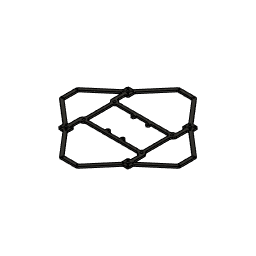
CarbonFiberBoard v13 (Autodesk Fusion 360 design; units mm, degrees)
Autodesk Fusion 360 part; units mm, degrees
sketch "草图1" plane through (0, 0, 0) normal (0, 0, 1) x (1, 0, 0)
  line L0 (42.5, 42.5) -> (-42.5, 42.5) construction
  line L1 (-42.5, 42.5) -> (-42.5, -42.5) construction
  line L2 (-42.5, -42.5) -> (42.5, -42.5) construction
  line L3 (42.5, -42.5) -> (42.5, 42.5) construction
  line L4 (42.5, 42.5) -> (-42.5, -42.5) construction
  line L5 (-42.5, 42.5) -> (42.5, -42.5) construction
  circle A0 centre (-42.5, 42.5) radius 2.25
  circle A1 centre (-45.682, 45.682) radius 1.05
  circle A2 centre (-45.682, 39.318) radius 1.05
  circle A3 centre (-39.318, 39.318) radius 1.05
  circle A4 centre (-39.318, 45.682) radius 1.05
  line L6 (0, 55) -> (0, -50) construction
  line L7 (-50, 0) -> (50, 0) construction
  circle A5 centre (45.682, 39.318) radius 1.05
  circle A6 centre (42.5, 42.5) radius 2.25
  circle A7 centre (39.318, 39.318) radius 1.05
  circle A8 centre (39.318, 45.682) radius 1.05
  circle A9 centre (45.682, 45.682) radius 1.05
  circle A10 centre (-45.682, -39.318) radius 1.05
  circle A11 centre (-45.682, -45.682) radius 1.05
  circle A12 centre (-42.5, -42.5) radius 2.25
  circle A13 centre (-39.318, -45.682) radius 1.05
  circle A14 centre (-39.318, -39.318) radius 1.05
  circle A15 centre (39.318, -45.682) radius 1.05
  circle A16 centre (45.682, -45.682) radius 1.05
  circle A17 centre (42.5, -42.5) radius 2.25
  circle A18 centre (39.318, -39.318) radius 1.05
  circle A19 centre (45.682, -39.318) radius 1.05
  line L8 (39.5, 21) -> (-39.5, 21) construction
  line L9 (-39.5, 21) -> (-39.5, -21) construction
  line L10 (-39.5, -21) -> (39.5, -21) construction
  line L11 (39.5, -21) -> (39.5, 21) construction
  line L12 (39.5, 21) -> (-39.5, -21) construction
  line L13 (-39.5, 21) -> (39.5, -21) construction
  circle A20 centre (-39.5, 21) radius 1.6
  circle A21 centre (39.5, 21) radius 1.6
  circle A22 centre (-39.5, -21) radius 1.6
  circle A23 centre (39.5, -21) radius 1.6
  line L14 (-35.9031, 22.75) -> (35.9031, 22.75)
  line L15 (-35.9031, 19.25) -> (35.9031, 19.25)
  line L16 (-41.25, 17.4031) -> (-41.25, -17.4031)
  line L17 (-37.75, 17.4031) -> (-37.75, -17.4031)
  line L18 (37.75, 17.4031) -> (37.75, -17.4031)
  line L19 (41.25, 17.4031) -> (41.25, -17.4031)
  line L20 (-35.9031, -19.25) -> (35.9031, -19.25)
  line L21 (-35.9031, -22.75) -> (35.9031, -22.75)
  line L22 (-40.5, 37) -> (-40.5, 24.873)
  line L23 (-42.7, 18.6) -> (-44.5, 21)
  line L24 (-44.5, 21) -> (-44.5, 37)
  line L25 (-38.5, 48) -> (-46.5, 48)
  line L26 (-48, 46.5) -> (-48, 38.5)
  line L27 (-37, 38.5) -> (-37, 46.5)
  line L28 (-37, 48) -> (-48, 37) construction
  line L29 (-48, 48) -> (-37, 37) construction
  arc A24 (-46.5, 48) -> (-48, 46.5) centre (-46.5, 46.5) ccw
  arc A25 (-48, 38.5) -> (-46.5, 37) centre (-46.5, 38.5) ccw
  arc A26 (-38.5, 37) -> (-37, 38.5) centre (-38.5, 38.5) ccw
  arc A27 (-37, 46.5) -> (-38.5, 48) centre (-38.5, 46.5) ccw
  line L30 (-46.5, 37) -> (-44.5, 37)
  line L31 (-40.5, 37) -> (-38.5, 37)
  arc A28 (-35.9031, 22.75) -> (-40.5, 24.873) centre (-39.5, 21) ccw
  arc A29 (-42.7, 18.6) -> (-41.25, 17.4031) centre (-39.5, 21) ccw
  arc A30 (48, 46.5) -> (46.5, 48) centre (46.5, 46.5) ccw
  line L32 (38.5, 48) -> (46.5, 48)
  arc A31 (38.5, 48) -> (37, 46.5) centre (38.5, 46.5) ccw
  line L33 (37, 38.5) -> (37, 46.5)
  line L34 (48, 46.5) -> (48, 38.5)
  arc A32 (46.5, 37) -> (48, 38.5) centre (46.5, 38.5) ccw
  line L35 (46.5, 37) -> (44.5, 37)
  line L36 (40.5, 37) -> (38.5, 37)
  arc A33 (37, 38.5) -> (38.5, 37) centre (38.5, 38.5) ccw
  line L37 (40.5, 37) -> (40.5, 24.873)
  line L38 (44.5, 21) -> (44.5, 37)
  line L39 (42.7, 18.6) -> (44.5, 21)
  line L40 (-46.5, -37) -> (-44.5, -37)
  arc A34 (-46.5, -37) -> (-48, -38.5) centre (-46.5, -38.5) ccw
  line L41 (-48, -46.5) -> (-48, -38.5)
  arc A35 (-48, -46.5) -> (-46.5, -48) centre (-46.5, -46.5) ccw
  line L42 (-38.5, -48) -> (-46.5, -48)
  arc A36 (-38.5, -48) -> (-37, -46.5) centre (-38.5, -46.5) ccw
  line L43 (-37, -38.5) -> (-37, -46.5)
  arc A37 (-37, -38.5) -> (-38.5, -37) centre (-38.5, -38.5) ccw
  line L44 (-40.5, -37) -> (-38.5, -37)
  line L45 (-40.5, -37) -> (-40.5, -24.873)
  line L46 (-44.5, -21) -> (-44.5, -37)
  line L47 (-42.7, -18.6) -> (-44.5, -21)
  line L48 (40.5, -37) -> (40.5, -24.873)
  line L49 (40.5, -37) -> (38.5, -37)
  arc A38 (38.5, -37) -> (37, -38.5) centre (38.5, -38.5) ccw
  line L50 (37, -38.5) -> (37, -46.5)
  arc A39 (37, -46.5) -> (38.5, -48) centre (38.5, -46.5) ccw
  line L51 (38.5, -48) -> (46.5, -48)
  arc A40 (46.5, -48) -> (48, -46.5) centre (46.5, -46.5) ccw
  line L52 (48, -46.5) -> (48, -38.5)
  arc A41 (48, -38.5) -> (46.5, -37) centre (46.5, -38.5) ccw
  line L53 (46.5, -37) -> (44.5, -37)
  line L54 (44.5, -21) -> (44.5, -37)
  line L55 (42.7, -18.6) -> (44.5, -21)
  arc A42 (41.25, 17.4031) -> (42.7, 18.6) centre (39.5, 21) ccw
  arc A43 (40.5, 24.873) -> (35.9031, 22.75) centre (39.5, 21) ccw
  arc A44 (-41.25, -17.4031) -> (-42.7, -18.6) centre (-39.5, -21) ccw
  arc A45 (-40.5, -24.873) -> (-35.9031, -22.75) centre (-39.5, -21) ccw
  arc A46 (35.9031, -22.75) -> (40.5, -24.873) centre (39.5, -21) ccw
  arc A47 (42.7, -18.6) -> (41.25, -17.4031) centre (39.5, -21) ccw
  arc A48 (37.75, -17.4031) -> (35.9031, -19.25) centre (39.5, -21) ccw
  arc A49 (35.9031, 19.25) -> (37.75, 17.4031) centre (39.5, 21) ccw
  arc A50 (-37.75, 17.4031) -> (-35.9031, 19.25) centre (-39.5, 21) ccw
  arc A51 (-35.9031, -19.25) -> (-37.75, -17.4031) centre (-39.5, -21) ccw
  point P0 (-42.5, 42.5)
  dimension "d1" = 85
  dimension "d2" = 85
  dimension "d3" = 4.5
  dimension "d4" = 2.1
  dimension "d5" = 4.5
  dimension "d7" = 360
  dimension "d9" = 79
  dimension "d10" = 42
  dimension "d11" = 3.2
  dimension "d12" = 8
  dimension "d13" = 8
  dimension "d14" = 8
  dimension "d15" = 8
  dimension "d16" = 3.5
  dimension "d17" = 3.5
  dimension "d18" = 2
  dimension "d19" = 2
  dimension "d20" = 11
  dimension "d21" = 11
  dimension "d22" = 1.5
  constraint horizontal L0
  constraint perpendicular L0 L1
  constraint parallel L0 L2
  constraint parallel L1 L3
  constraint coincident L4 origin
  constraint coincident L5 origin
  constraint coincident P0 L0.end
  constraint coincident L5 A1.centre
  constraint vertical L6
  constraint horizontal L7
  constraint symmetric A0 L6 A6
  constraint symmetric A1 L6 A9
  constraint symmetric A2 L6 A5
  constraint symmetric A3 L6 A7
  constraint symmetric A4 L6 A8
  constraint symmetric A0 L7 A12
  constraint symmetric A1 L7 A11
  constraint symmetric A2 L7 A10
  constraint symmetric A3 L7 A14
  constraint symmetric A4 L7 A13
  constraint symmetric L7 A5 A19
  constraint symmetric L7 A6 A17
  constraint symmetric L7 A7 A18
  constraint symmetric L7 A8 A15
  constraint symmetric L7 A9 A16
  constraint horizontal L8
  constraint perpendicular L8 L9
  constraint parallel L8 L10
  constraint parallel L9 L11
  constraint coincident L12 origin
  constraint coincident L13 origin
  constraint coincident L8.end L9.start
  constraint symmetric L6 A20 A21
  constraint symmetric L7 A20 A22
  constraint symmetric L7 A21 A23
  constraint concentric A20 A28
  constraint concentric A21 A42
  constraint concentric A22 A44
  constraint concentric A23 A46
  constraint parallel L8 L14
  constraint coincident L15.start A28
  constraint coincident L15.end A42
  constraint parallel L8 L15
  constraint symmetric L8 L14 L15
  constraint parallel L9 L16
  constraint coincident L17.start A28
  constraint parallel L9 L17
  constraint symmetric L6 L16.start L19.start
  constraint symmetric L6 L16.end L19.end
  constraint symmetric L6 L17.start L18.start
  constraint symmetric L6 L17.end L18.end
  constraint symmetric L7 L14.start L21.start
  constraint symmetric L7 L14.end L21.end
  constraint symmetric L7 L15.start L20.start
  constraint symmetric L7 L15.end L20.end
  constraint vertical L22
  constraint coincident L23.start A28
  constraint vertical L24
  constraint tangent L23 A28
  constraint horizontal L25
  constraint perpendicular L25 L26
  constraint parallel L25 L30
  constraint parallel L26 L27
  constraint coincident L28 P0
  constraint coincident L29 P0
  constraint coincident L29.start L26
  constraint coincident L29.start L25
  constraint tangent L26 A24
  constraint tangent L25 A24
  constraint coincident L28.end L26
  constraint coincident L28.end L30
  constraint tangent L26 A25
  constraint tangent A25 L30
  constraint equal A24 A25
  constraint coincident L29.end L30
  constraint coincident L29.end L27
  constraint tangent A26 L30
  constraint tangent L27 A26
  constraint equal A24 A26
  constraint coincident L28.start L27
  constraint coincident L28.start L25
  constraint tangent L27 A27
  constraint tangent L25 A27
  constraint equal A24 A27
  constraint coincident L22.start L30
  constraint collinear L30 L31
  constraint concentric A28 A29
  constraint symmetric L6 L22.start L36.start
  constraint symmetric L6 L22.end L37.end
  constraint symmetric L6 L23.start L39.start
  constraint symmetric L6 L23.end L38.start
  constraint symmetric L6 L24.end L35.end
  constraint symmetric L6 L26.start A30.start
  constraint symmetric L6 L25.end A30.end
  constraint symmetric L6 A24 A30
  constraint symmetric L6 L26.end L34.end
  constraint symmetric L6 A25.end A32.start
  constraint symmetric L6 A25 A32
  constraint symmetric L6 A26.start L36.end
  constraint symmetric L6 L27.start L33.start
  constraint symmetric L6 A26 A33
  constraint symmetric L6 L27.end A31.end
  constraint symmetric L6 L25.start L32.start
  constraint symmetric L6 A27 A31
  constraint symmetric L7 L22.start L44.start
  constraint symmetric L7 L22.end L45.end
  constraint symmetric L7 L23.start L47.start
  constraint symmetric L7 L23.end L46.start
  constraint symmetric L7 L24.end L40.end
  constraint symmetric L7 L26.start L41.start
  constraint symmetric L7 L25.end A35.end
  constraint symmetric L7 A24 A35
  constraint symmetric L7 L26.end A34.end
  constraint symmetric L7 A25.end L40.start
  constraint symmetric L7 A25 A34
  constraint symmetric L7 A26.start A37.end
  constraint symmetric L7 L27.start L43.start
  constraint symmetric L7 A26 A37
  constraint symmetric L7 L27.end A36.end
  constraint symmetric L7 L25.start L42.start
  constraint symmetric L7 A27 A36
  constraint symmetric L7 A30.end L51.end
  constraint symmetric L7 A30.start A40.end
  constraint symmetric L7 A30 A40
  constraint symmetric L7 L32.start A39.end
  constraint symmetric L7 A31.end L50.end
  constraint symmetric L7 A31 A39
  constraint symmetric L7 L33.start A38.end
  constraint symmetric L7 L34.end L52.end
  constraint symmetric L7 A32.start A41.end
  constraint symmetric L7 A32 A41
  constraint symmetric L7 L35.end L53.end
  constraint symmetric L7 L36.start L48.start
  constraint symmetric L7 L36.end L49.end
  constraint symmetric L7 A33 A38
  constraint symmetric L7 L37.end L48.end
  constraint symmetric L7 L38.start L54.start
  constraint symmetric L7 L39.start L55.start
  constraint concentric A42 A43
  constraint concentric A44 A45
  constraint concentric A46 A47
  constraint coincident L10.end L11.start
  constraint coincident L8.start L11.end
  constraint coincident L9.end L10.start
  measures "d1" distance of L0.start P0
  measures "d2" distance of L0 L2
  measures "d3" diameter of A0
  measures "d4" diameter of A1
  measures "d5" distance of P0 A1.centre
  measures "d9" distance of L8.start L8.end
  measures "d10" distance of L8 L10
  measures "d11" diameter of A20
  measures "d12" diameter of A28
  measures "d13" diameter of A42
  measures "d14" diameter of A44
  measures "d15" diameter of A46
  measures "d16" distance of L14 L15
  measures "d17" distance of L16 L17
  measures "d18" distance of L1 L22
  measures "d19" distance of L1 L24
  measures "d20" distance of L26 L27
  measures "d21" distance of L25 L30
  measures "d22" radius of A24
extrude "拉伸1" add sketch "草图1" along normal blind 2
fillet "圆角1" radius 1 8 edges at (-44.5, -37, 1) (-40.5, -37, 1) (44.5, -37, 1) (40.5, -37, 1) (-44.5, 37, 1) (40.5, 37, 1) (44.5, 37, 1) (-40.5, 37, 1)
fillet "圆角2" radius 3 4 edges at (-44.5, 21, 1) (-44.5, -21, 1) (44.5, -21, 1) (44.5, 21, 1)
fillet "圆角3" radius 3 4 edges at (41.25, -17.4031, 1) (41.25, 17.4031, 1) (-41.25, -17.4031, 1) (-41.25, 17.4031, 1)
fillet "圆角4" radius 2 4 edges at (-40.5, -24.873, 1) (-40.5, 24.873, 1) (40.5, 24.873, 1) (40.5, -24.873, 1)
fillet "圆角5" radius 2 4 edges at (35.9031, -22.75, 1) (-35.9031, -22.75, 1) (-35.9031, 22.75, 1) (35.9031, 22.75, 1)
sketch "草图3" plane through (0, 0, 0) normal (0, 0, 1) x (1, 0, 0)
  line L0 (10, 17.5) -> (-10, 17.5) construction
  line L1 (-10, 17.5) -> (-10, -17.5) construction
  line L2 (-10, -17.5) -> (10, -17.5) construction
  line L3 (10, -17.5) -> (10, 17.5) construction
  line L4 (10, 17.5) -> (-10, -17.5) construction
  line L5 (-10, 17.5) -> (10, -17.5) construction
  circle A0 centre (-10, 17.5) radius 1
  circle A1 centre (10, 17.5) radius 1
  circle A2 centre (-10, -17.5) radius 1
  circle A3 centre (10, -17.5) radius 1
  line L6 (-7.5, 17.5) -> (-7.5, 19.5)
  arc A4 (-7.5, 19.5) -> (-12.5, 19.5) centre (-10, 19.5) ccw
  line L7 (-12.5, 19.5) -> (-12.5, 17.5)
  arc A5 (-12.5, 17.5) -> (-7.5, 17.5) centre (-10, 17.5) ccw
  line L8 (-10, 17.5) -> (-10, 19.5) construction
  line L9 (0, 0) -> (0, 8.2439) construction
  line L10 (0, 0) -> (4, 0) construction
  arc A6 (7.5, 17.5) -> (12.5, 17.5) centre (10, 17.5) ccw
  line L11 (12.5, 19.5) -> (12.5, 17.5)
  arc A7 (12.5, 19.5) -> (7.5, 19.5) centre (10, 19.5) ccw
  line L12 (7.5, 17.5) -> (7.5, 19.5)
  arc A8 (-7.5, -17.5) -> (-12.5, -17.5) centre (-10, -17.5) ccw
  line L13 (-12.5, -19.5) -> (-12.5, -17.5)
  arc A9 (-12.5, -19.5) -> (-7.5, -19.5) centre (-10, -19.5) ccw
  line L14 (-7.5, -17.5) -> (-7.5, -19.5)
  line L15 (7.5, -17.5) -> (7.5, -19.5)
  arc A10 (7.5, -19.5) -> (12.5, -19.5) centre (10, -19.5) ccw
  line L16 (12.5, -19.5) -> (12.5, -17.5)
  arc A11 (12.5, -17.5) -> (7.5, -17.5) centre (10, -17.5) ccw
  dimension "d50" = 20
  dimension "d51" = 35
  dimension "d52" = 2
  dimension "d53" = 2
  dimension "d54" = 2
  dimension "d55" = 2
  dimension "d56" = 5
  dimension "d57" = 2
  constraint horizontal L0
  constraint perpendicular L0 L1
  constraint parallel L0 L2
  constraint parallel L1 L3
  constraint coincident L4 L9.start
  constraint coincident L5 L9.start
  constraint coincident L9.start L10.start
  constraint coincident L0.end L1.start
  constraint coincident L0.start L3.end
  constraint coincident L1.end L2.start
  constraint coincident L2.end L3.start
  constraint tangent L6 A4
  constraint tangent A4 L7
  constraint parallel L6 L7
  constraint tangent L7 A5
  constraint tangent L6 A5
  constraint parallel L1 L8
  constraint parallel L3 L9
  constraint perpendicular L9 L10
  constraint symmetric L6.start L9 A6.start
  constraint symmetric L6.end L9 A7.end
  constraint symmetric A4.end L9 L11.start
  constraint symmetric L7.end L9 A6.end
  constraint symmetric A4 L9 A7
  constraint symmetric A5 L9 A6
  constraint symmetric L6.start L10 A8.start
  constraint symmetric L6.end L10 A9.end
  constraint symmetric A4.end L10 L13.start
  constraint symmetric L7.end L10 A8.end
  constraint symmetric A4 L10 A9
  constraint symmetric A5 L10 A8
  constraint symmetric L10 A6.end L16.end
  constraint symmetric L10 A6.start L15.start
  constraint symmetric L10 A6 A11
  constraint symmetric L10 L11.start A10.end
  constraint symmetric L10 A7.end L15.end
  constraint symmetric L10 A7 A10
  measures "d50" distance of L1 L3
  measures "d51" distance of L0 L2
  measures "d52" diameter of A0
  measures "d53" diameter of A1
  measures "d54" diameter of A2
  measures "d55" diameter of A3
  measures "d56" distance of L6 L7
  measures "d57" distance of L0.end A4.centre
extrude "拉伸3" add sketch "草图3" along normal blind 2
sketch "草图5" plane through (0, 0, 2) normal (0, 0, 1) x (-1, 0, 0)
  circle A0 centre (-10, 17.5) radius 1
  line L0 (-7.5, 19.25) -> (7.5, 19.25)
  line L1 (7.5, 19.25) -> (7.5, 17.5)
  arc A1 (7.5, 17.5) -> (12.5, 17.5) centre (10, 17.5) ccw
  line L2 (12.5, 17.5) -> (12.5, 19.25)
  line L3 (12.5, 19.25) -> (35.9031, 19.25)
  arc A2 (35.9031, 19.25) -> (37.75, 17.4031) centre (39.5, 21) ccw
  line L4 (37.75, 17.4031) -> (37.75, -17.4031)
  arc A3 (37.75, -17.4031) -> (35.9031, -19.25) centre (39.5, -21) ccw
  line L5 (35.9031, -19.25) -> (12.5, -19.25)
  line L6 (12.5, -19.25) -> (12.5, -17.5)
  arc A4 (12.5, -17.5) -> (7.5, -17.5) centre (10, -17.5) ccw
  line L7 (7.5, -17.5) -> (7.5, -19.25)
  line L8 (7.5, -19.25) -> (-7.5, -19.25)
  line L9 (-7.5, -19.25) -> (-7.5, -17.5)
  arc A5 (-7.5, -17.5) -> (-12.5, -17.5) centre (-10, -17.5) ccw
  line L10 (-12.5, -17.5) -> (-12.5, -19.25)
  line L11 (-12.5, -19.25) -> (-35.9031, -19.25)
  arc A6 (-35.9031, -19.25) -> (-37.75, -17.4031) centre (-39.5, -21) ccw
  line L12 (-37.75, -17.4031) -> (-37.75, 17.4031)
  arc A7 (-37.75, 17.4031) -> (-35.9031, 19.25) centre (-39.5, 21) ccw
  line L13 (-35.9031, 19.25) -> (-12.5, 19.25)
  line L14 (-12.5, 19.25) -> (-12.5, 17.5)
  arc A8 (-12.5, 17.5) -> (-7.5, 17.5) centre (-10, 17.5) ccw
  line L15 (-7.5, 17.5) -> (-7.5, 19.25)
  circle A9 centre (10, -17.5) radius 1
  circle A10 centre (10, 17.5) radius 1
  circle A11 centre (-10, -17.5) radius 1
  circle A12 centre (39.318, -45.682) radius 1.05
  circle A13 centre (-45.682, -39.318) radius 1.05
  circle A14 centre (45.682, 39.318) radius 1.05
  circle A15 centre (45.682, 45.682) radius 1.05
  circle A16 centre (42.5, 42.5) radius 2.25
  circle A17 centre (39.318, 45.682) radius 1.05
  circle A18 centre (39.318, 39.318) radius 1.05
  circle A19 centre (45.682, -45.682) radius 1.05
  circle A20 centre (-39.318, -45.682) radius 1.05
  circle A21 centre (-39.318, -39.318) radius 1.05
  circle A22 centre (42.5, -42.5) radius 2.25
  circle A23 centre (45.682, -39.318) radius 1.05
  circle A24 centre (39.318, -39.318) radius 1.05
  circle A25 centre (-42.5, -42.5) radius 2.25
  circle A26 centre (-45.682, -45.682) radius 1.05
  circle A27 centre (39.5, 21) radius 1.6
  circle A28 centre (-39.5, 21) radius 1.6
  circle A29 centre (39.5, -21) radius 1.6
  circle A30 centre (-39.5, -21) radius 1.6
  circle A31 centre (-45.682, 39.318) radius 1.05
  circle A32 centre (-39.318, 39.318) radius 1.05
  circle A33 centre (-39.318, 45.682) radius 1.05
  circle A34 centre (-45.682, 45.682) radius 1.05
  circle A35 centre (-42.5, 42.5) radius 2.25
  arc A36 (-43.9, -20.2) -> (-44.5, -22) centre (-41.5, -22) ccw
  line L16 (-44.5, -22) -> (-44.5, -36)
  arc A37 (-45.5, -37) -> (-44.5, -36) centre (-45.5, -36) ccw
  line L17 (-45.5, -37) -> (-46.5, -37)
  arc A38 (-46.5, -37) -> (-48, -38.5) centre (-46.5, -38.5) ccw
  line L18 (-48, -38.5) -> (-48, -46.5)
  arc A39 (-48, -46.5) -> (-46.5, -48) centre (-46.5, -46.5) ccw
  line L19 (-46.5, -48) -> (-38.5, -48)
  arc A40 (-38.5, -48) -> (-37, -46.5) centre (-38.5, -46.5) ccw
  line L20 (-37, -46.5) -> (-37, -38.5)
  arc A41 (-37, -38.5) -> (-38.5, -37) centre (-38.5, -38.5) ccw
  line L21 (-38.5, -37) -> (-39.5, -37)
  arc A42 (-40.5, -36) -> (-39.5, -37) centre (-39.5, -36) ccw
  line L22 (-40.5, -36) -> (-40.5, -26.9161)
  arc A43 (-38.8333, -24.9441) -> (-40.5, -26.9161) centre (-38.5, -26.9161) ccw
  arc A44 (-38.8333, -24.9441) -> (-36.3775, -23.5) centre (-39.5, -21) ccw
  arc A45 (-34.8163, -22.75) -> (-36.3775, -23.5) centre (-34.8163, -24.75) ccw
  line L23 (-34.8163, -22.75) -> (34.8163, -22.75)
  arc A46 (36.3775, -23.5) -> (34.8163, -22.75) centre (34.8163, -24.75) ccw
  arc A47 (36.3775, -23.5) -> (38.8333, -24.9441) centre (39.5, -21) ccw
  arc A48 (40.5, -26.9161) -> (38.8333, -24.9441) centre (38.5, -26.9161) ccw
  line L24 (40.5, -26.9161) -> (40.5, -36)
  arc A49 (39.5, -37) -> (40.5, -36) centre (39.5, -36) ccw
  line L25 (39.5, -37) -> (38.5, -37)
  arc A50 (38.5, -37) -> (37, -38.5) centre (38.5, -38.5) ccw
  line L26 (37, -38.5) -> (37, -46.5)
  arc A51 (37, -46.5) -> (38.5, -48) centre (38.5, -46.5) ccw
  line L27 (38.5, -48) -> (46.5, -48)
  arc A52 (46.5, -48) -> (48, -46.5) centre (46.5, -46.5) ccw
  line L28 (48, -46.5) -> (48, -38.5)
  arc A53 (48, -38.5) -> (46.5, -37) centre (46.5, -38.5) ccw
  line L29 (46.5, -37) -> (45.5, -37)
  arc A54 (44.5, -36) -> (45.5, -37) centre (45.5, -36) ccw
  line L30 (44.5, -36) -> (44.5, -22)
  arc A55 (44.5, -22) -> (43.9, -20.2) centre (41.5, -22) ccw
  line L31 (43.9, -20.2) -> (42.7, -18.6)
  arc A56 (42.7, -18.6) -> (42.2143, -18.0619) centre (39.5, -21) ccw
  arc A57 (41.25, -15.8583) -> (42.2143, -18.0619) centre (44.25, -15.8583) ccw
  line L32 (41.25, -15.8583) -> (41.25, 15.8583)
  arc A58 (42.2143, 18.0619) -> (41.25, 15.8583) centre (44.25, 15.8583) ccw
  arc A59 (42.2143, 18.0619) -> (42.7, 18.6) centre (39.5, 21) ccw
  line L33 (42.7, 18.6) -> (43.9, 20.2)
  arc A60 (43.9, 20.2) -> (44.5, 22) centre (41.5, 22) ccw
  line L34 (44.5, 22) -> (44.5, 36)
  arc A61 (45.5, 37) -> (44.5, 36) centre (45.5, 36) ccw
  line L35 (45.5, 37) -> (46.5, 37)
  arc A62 (46.5, 37) -> (48, 38.5) centre (46.5, 38.5) ccw
  line L36 (48, 38.5) -> (48, 46.5)
  arc A63 (48, 46.5) -> (46.5, 48) centre (46.5, 46.5) ccw
  line L37 (46.5, 48) -> (38.5, 48)
  arc A64 (38.5, 48) -> (37, 46.5) centre (38.5, 46.5) ccw
  line L38 (37, 46.5) -> (37, 38.5)
  arc A65 (37, 38.5) -> (38.5, 37) centre (38.5, 38.5) ccw
  line L39 (38.5, 37) -> (39.5, 37)
  arc A66 (40.5, 36) -> (39.5, 37) centre (39.5, 36) ccw
  line L40 (40.5, 36) -> (40.5, 26.9161)
  arc A67 (38.8333, 24.9441) -> (40.5, 26.9161) centre (38.5, 26.9161) ccw
  arc A68 (38.8333, 24.9441) -> (36.3775, 23.5) centre (39.5, 21) ccw
  arc A69 (34.8163, 22.75) -> (36.3775, 23.5) centre (34.8163, 24.75) ccw
  line L41 (34.8163, 22.75) -> (-34.8163, 22.75)
  arc A70 (-36.3775, 23.5) -> (-34.8163, 22.75) centre (-34.8163, 24.75) ccw
  arc A71 (-36.3775, 23.5) -> (-38.8333, 24.9441) centre (-39.5, 21) ccw
  arc A72 (-40.5, 26.9161) -> (-38.8333, 24.9441) centre (-38.5, 26.9161) ccw
  line L42 (-40.5, 26.9161) -> (-40.5, 36)
  arc A73 (-39.5, 37) -> (-40.5, 36) centre (-39.5, 36) ccw
  line L43 (-39.5, 37) -> (-38.5, 37)
  arc A74 (-38.5, 37) -> (-37, 38.5) centre (-38.5, 38.5) ccw
  line L44 (-37, 38.5) -> (-37, 46.5)
  arc A75 (-37, 46.5) -> (-38.5, 48) centre (-38.5, 46.5) ccw
  line L45 (-38.5, 48) -> (-46.5, 48)
  arc A76 (-46.5, 48) -> (-48, 46.5) centre (-46.5, 46.5) ccw
  line L46 (-48, 46.5) -> (-48, 38.5)
  arc A77 (-48, 38.5) -> (-46.5, 37) centre (-46.5, 38.5) ccw
  line L47 (-46.5, 37) -> (-45.5, 37)
  arc A78 (-44.5, 36) -> (-45.5, 37) centre (-45.5, 36) ccw
  line L48 (-44.5, 36) -> (-44.5, 22)
  arc A79 (-44.5, 22) -> (-43.9, 20.2) centre (-41.5, 22) ccw
  line L49 (-43.9, 20.2) -> (-42.7, 18.6)
  arc A80 (-42.7, 18.6) -> (-42.2143, 18.0619) centre (-39.5, 21) ccw
  arc A81 (-41.25, 15.8583) -> (-42.2143, 18.0619) centre (-44.25, 15.8583) ccw
  line L50 (-41.25, 15.8583) -> (-41.25, -15.8583)
  arc A82 (-42.2143, -18.0619) -> (-41.25, -15.8583) centre (-44.25, -15.8583) ccw
  arc A83 (-42.2143, -18.0619) -> (-42.7, -18.6) centre (-39.5, -21) ccw
  line L51 (-42.7, -18.6) -> (-43.9, -20.2)
  circle A84 centre (42.5, -42.5) radius 32.5 construction
  circle A85 centre (-42.5, -42.5) radius 32.5 construction
  circle A86 centre (42.5, 42.5) radius 32.5 construction
  circle A87 centre (-42.5, 42.5) radius 32.5 construction
  line L52 (7.5, 60) -> (7.5, 75) construction
  arc A88 (7.5, 75) -> (-7.5, 75) centre (0, 75) ccw construction
  line L53 (-7.5, 75) -> (-7.5, 60) construction
  arc A89 (-7.5, 60) -> (7.5, 60) centre (0, 60) ccw construction
  line L54 (0, 60) -> (0, 75) construction
  circle A90 centre (10, 80) radius 1.05
  line L55 (37, 46.5) -> (10, 78)
  line L56 (10, 78) -> (0, 78)
  line L57 (40.9826, 48) -> (11.8397, 82)
  line L58 (11.8397, 82) -> (0, 82)
  line L59 (40.9826, 48) -> (37, 46.5)
  line L60 (-40.9826, 48) -> (-37, 46.5)
  line L61 (-40.9826, 48) -> (-11.8397, 82)
  line L62 (-37, 46.5) -> (-10, 78)
  line L63 (-10, 78) -> (0, 78)
  line L64 (-11.8397, 82) -> (0, 82)
  circle A91 centre (-10, 80) radius 1.05
  line L65 (-48, 40.9826) -> (-46.5, 37)
  line L66 (-48, 40.9826) -> (-82, 11.8397)
  line L67 (-46.5, 37) -> (-78, 10)
  line L68 (-82, 11.8397) -> (-82, 0)
  circle A92 centre (-80, 10) radius 1.05
  line L69 (-78, 10) -> (-78, 0)
  line L70 (-78, -10) -> (-78, 0)
  line L71 (-82, -11.8397) -> (-82, 0)
  line L72 (-48, -40.9826) -> (-82, -11.8397)
  line L73 (-46.5, -37) -> (-78, -10)
  line L74 (-48, -40.9826) -> (-46.5, -37)
  circle A93 centre (-80, -10) radius 1.05
  line L75 (-40.9826, -48) -> (-37, -46.5)
  line L76 (-40.9826, -48) -> (-11.8397, -82)
  line L77 (-37, -46.5) -> (-10, -78)
  line L78 (-11.8397, -82) -> (0, -82)
  circle A94 centre (-10, -80) radius 1.05
  line L79 (-10, -78) -> (0, -78)
  line L80 (10, -78) -> (0, -78)
  line L81 (11.8397, -82) -> (0, -82)
  line L82 (40.9826, -48) -> (11.8397, -82)
  line L83 (37, -46.5) -> (10, -78)
  line L84 (40.9826, -48) -> (37, -46.5)
  circle A95 centre (10, -80) radius 1.05
  line L85 (48, -40.9826) -> (46.5, -37)
  line L86 (48, -40.9826) -> (82, -11.8397)
  line L87 (46.5, -37) -> (78, -10)
  line L88 (82, -11.8397) -> (82, 0)
  circle A96 centre (80, -10) radius 1.05
  line L89 (78, -10) -> (78, 0)
  line L90 (78, 10) -> (78, 0)
  line L91 (82, 11.8397) -> (82, 0)
  line L92 (48, 40.9826) -> (82, 11.8397)
  line L93 (46.5, 37) -> (78, 10)
  line L94 (48, 40.9826) -> (46.5, 37)
  circle A97 centre (80, 10) radius 1.05
  dimension "d60" = 65
  dimension "d61" = 65
  dimension "d62" = 65
  dimension "d63" = 65
  dimension "d64" = 15
  dimension "d65" = 15
  dimension "d66" = 60
  dimension "d67" = 2.1
  dimension "d68" = 5
  dimension "d69" = 10
  dimension "d70" = 4
  dimension "d71" = 2
  dimension "d72" = 2
  dimension "d74" = 360
  constraint concentric A22 A84
  constraint concentric A25 A85
  constraint concentric A16 A86
  constraint concentric A35 A87
  constraint tangent L52 A88
  constraint tangent A88 L53
  constraint parallel L52 L53
  constraint tangent L53 A89
  constraint tangent L52 A89
  constraint vertical L54
  constraint vertical origin A89.centre
  constraint coincident A64.end L38.start
  constraint coincident L54 L56.end
  constraint perpendicular L54 L56
  constraint coincident L37 L57.start
  constraint horizontal L58
  constraint parallel L55 L57
  constraint vertical A90.centre L55.end
  constraint symmetric L54 A90 A91
  constraint symmetric L54 A64.end L44.end
  constraint symmetric L54 L55.end L62.end
  constraint symmetric L54 L56.end L63.end
  constraint symmetric L54 L57.start L60.start
  constraint symmetric L54 L57.end L61.end
  constraint symmetric L54 L58.end L64.end
  constraint vertical L58.end L56.end
  measures "d60" diameter of A84
  measures "d61" diameter of A85
  measures "d62" diameter of A87
  measures "d63" diameter of A86
  measures "d64" distance of L52 L53
  measures "d65" distance of A89.centre A88.centre
  measures "d66" distance of origin A89.centre
  measures "d67" diameter of A90
  measures "d68" vertical distance of A88.centre A90.centre
  measures "d69" horizontal distance of A88.centre A90.centre
  measures "d70" distance of L55 L57
  measures "d71" distance of A90.centre L56
  measures "d72" distance of A90.centre L58
extrude "拉伸4" add sketch "草图5" against normal blind 2 contours A38 L18 L46 A77 L66 L67 L68 L69 L70 L71 L72 L73 | L19 A40 A51 L27 L76 L77 L78 L79 L80 L81 L82 L83 | L37 A64 A75 L45 L55 L56 L57 L58 L61 L62 L63 L64 | L28 A53 A62 L36 L86 L87 L88 L89 L90 L91 L92 L93
fillet "圆角7" radius 2 8 edges at (-78, 10, 1) (-10, 78, 1) (10, 78, 1) (78, 10, 1) (78, -10, 1) (10, -78, 1) (-10, -78, 1) (-78, -10, 1)
fillet "圆角7" radius 2 16 edges at (-11.8397, -82, 1) (11.8397, -82, 1) (40.9826, -48, 1) (48, -40.9826, 1) (82, -11.8397, 1) (82, 11.8397, 1) (48, 40.9826, 1) (40.9826, 48, 1) (11.8397, 82, 1) (-11.8397, 82, 1) (-40.9826, 48, 1) (-48, 40.9826, 1) (-82, 11.8397, 1) (-82, -11.8397, 1) (-48, -40.9826, 1) (-40.9826, -48, 1)
fillet "圆角7" radius 2 8 edges at (37, 46.5, 1) (-37, 46.5, 1) (-46.5, 37, 1) (-46.5, -37, 1) (-37, -46.5, 1) (37, -46.5, 1) (46.5, -37, 1) (46.5, 37, 1)
